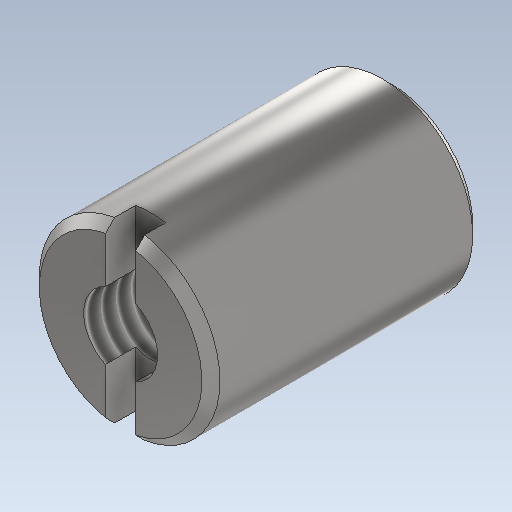
# Autodesk Inventor part: ARU-309S
Saved by Autodesk Inventor 2020.4 (Build 244396000, 396)
## iProperties
Created: 2021-08-03
Part Number: ARU-309S
Material: ステンレス鋼 AISI 304
Document SubType Name: Modeling
Designer: naoki
Density: 8 g/cm^3
Appearance: 半つや出し
Mass: 1.78344 g
Surface Area: 3.09379 cm^2
Volume: 0.230121 cm^3
Description: 既製品
Author: naoki
Title: ARU-309_5S
Autodesk Inventor part; units mm, degrees
ref_plane "YZ Plane" through (0, 0, 0) normal (1, 0, 0) x (0, 1, 0)
ref_plane "XZ Plane" through (0, 0, 0) normal (0, 1, 0) x (-1, 0, 0)
ref_plane "XY Plane" through (0, 0, 0) normal (0, 0, 1) x (1, 0, 0)
sketch "スケッチ1" plane through (0, 0, 0) normal (0, 1, 0) x (-1, 0, 0)
  line L0 (0, 0) -> (9, 0)
  line L1 (9, 0) -> (9, -3)
  line L2 (9, -3) -> (0, -3)
  line L3 (0, -3) -> (0, 0)
  dimension "d0" = 9
  dimension "d1" = 3
  constraints: 8 end point, 2 parallel, 1 horizontal, 1 perpendicular
  measures "d0" distance of L1.end L2.end
  measures "d1" distance of L0.end L1.end
revolve "回転1" add sketch "スケッチ1" angle 360 about axis through (0, 0, 0) along (-1, 0, 0)
sketch "スケッチ2" plane through (0, 0, 0) normal (1, 0, 0) x (0, 0, -1)
  point P0 (0, 0)
  point P1 (0, 0)
  constraints: 1 coincident
hole "穴1" at (0, 0, 0) direction (-1, 0, 0) diameter 2.459 end through all thread size "M3x0.5" class "6H" standard "ANSI Metric M Profile"
sketch "スケッチ3" plane through (0, 0, 0) normal (1, 0, 0) x (0, 0, -1)
  circle A0 centre (0, 0) radius 3 projected
  line L0 (3, 0) -> (-3, 0)
  line L1 (3, -0.5) -> (-3, -0.5)
  line L2 (3, 0.5) -> (-3, 0.5)
  line L3 (3, 0.5) -> (3, -0.5)
  line L4 (-3, 0.5) -> (-3, -0.5)
  point P0 (-2.958, -0.5)
  point P1 (2.958, -0.5)
  point P2 (2.958, 0.5)
  point P3 (-2.958, 0.5)
  dimension "d10" = 0.5
  constraints: 10 end point, 2 parallel, 2 point on circle, 2 symmetric about line, 1 horizontal, 1 perpendicular
  measures "d10" distance between parallel lines of L0 L1
extrude "押し出し1" cut sketch "スケッチ3" against normal blind 1 contours L0 A0 L2 | A0 L1 L0
chamfer "面取り1" distance 0.3 angle 45 3 edges at (-9, 0, 3) (0, 3, 0) (0, -3, 0)
